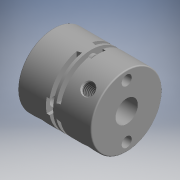
# Autodesk Inventor part: MCGS16-5-8_b
Saved by Autodesk Inventor 2017.3 (Build 213256000, 256)
## iProperties
Part Number: MCGS16-5-8_b
Material: Generic
Catalog Web Link: www.cadenas.de
Description: MCGS, MCGSLK, MCGSRK, MCGSWK_BODY-Couplings - Standard Torque, Set Screw Type - Single Disk Type
Vendor: MISUMI
Document SubType Name: Modeling
Designer: partserver
Manufacturer: MISUMI
Mass: 2.26083 g
Surface Area: 22.403 cm^2
Volume: 2.26083 cm^3
Density: 1 g/cm^3
Appearance: PSOLRGB-192-192-192
Category: PARTsolutions
Company: MISUMI
Title: MCGS16-5-8
Author: Cadenas PARTsolutions
Comments: Couplings - Standard Torque, Set Screw Type - Single Disk Type
PSOL_IDENT_0: {$CADENAS_DATA\23d-libs\misumi\metric\50_couplings\mcgs.prj},241 {VTYP=3D},{NB=MCGS16-5-8_b},{LINA=M
PSOL_IDENT_1: CGS16-5-8},{NN=MCGS, MCGSLK, MCGSRK, MCGSWK_BODY},{DATE=08.06.2021 06:32:33},{GEOMDATE=28.08.2013 00
PSOL_IDENT_2: :00:00},{VERSION=},{LINEID=1040},{WBVAR=HS,KGHS,DD1,ALT1,LDC,DD2,ALT2,RDC,ALT3,ALT4},{WBNUMERIC=LDC,
PSOL_IDENT_3: RDC}  {NB=MCGS16-5-8_b},{LINA=MCGS16-5-8},{KT=DUMMY},{PN=MCGS16-5-8},{HS=MCGS},{HSALG='MCGS','Standa
PSOL_IDENT_4: rd Hole','','Key Groove Hole'},{KGHS=},{KGHSALG='','N/A'},{MATB=Aluminum Die Casting},{MATD=Polyimid
PSOL_IDENT_5: },{STB=Electroless Nickel Plating},{AC=Set Screw},{D=16},{DDIA=16.000},{D1='4','4','5','5','6','6','
PSOL_IDENT_6: 6.35','6.35','7','7','8','8'},{DD1=5},{DD1ALG1='4','4','5','5','6','6','6.35','6.35','7','7','8','8'
PSOL_IDENT_7: },{DD1ALG2=5},{ALT1=},{ALT1ALG=},{LDC=0.0},{LDCALG=0},{LDCALG1=},{LK=0},{D2='5','5','6','6','6.35','
PSOL_IDENT_8: 6.35','7','7','8','8'},{DD2=8},{DDD1=0},{DD2ALG1='5','5','6','6','6.35','6.35','7','7','8','8'},{DD2
PSOL_IDENT_9: ALG11='4','4','5','5','6','6','6.35','6.35','7','7','8','8'},{DD2ALG2=8},{ALT2=},{ALT2ALG=},{RDC=0.0
PSOL_IDENT_10: },{RDCALG=0},{RDCALG1=},{RK=0},{DD3=6.8},{L=16.5},{L1=16.500},{LL=7},{LL1=7.000},{F=3},{F1=3.000},{M=
PSOL_IDENT_11: M3},{T=0.7},{NO=3},{DDIA2=11.2014},{SC1=1.7500},{SC2=6.0000},{DL=5},{TSIMD=3.000},{DR=8},{TSIMIN=2.4
PSOL_IDENT_12: 59},{ALTALG2='','Select RDC'},{TSI=M3},{R1=2.250},{DDIA3=12.000},{LL2=0.950},{C=3.000},{B=3.500},{E=
PSOL_IDENT_13: 3.200},{F2=0.650},{LL3=4.400},{DDIA4=9.000},{TSIMD1=4.800},{TTL=0.0},{TTR=0.0},{ALT3=},{ALT3ALG= '',
PSOL_IDENT_14: 'N/A'},{ALT3PN=},{ALT4=},{ALT4ALG= '', 'N/A'},{ALT4PN=},{KLH=0},{KRH=2},{TTKLH=0.0},{TTKRH=1.0},{MS
PSOL_IDENT_15: S=3},{LSS=4},{DID=7.6}
NB: MCGS16-5-8_b
NN: MCGS, MCGSLK, MCGSRK, MCGSWK_BODY
NT: Couplings - Standard Torque, Set Screw Type - Single Disk Type
NBSYN: $PN._b
LINA: MCGS16-5-8
CATALOG: Misumi
PN: MCGS16-5-8
HS: Standard Hole
KGHS: N/A
MATB: Aluminum Die Casting
MATD: Polyimid
STB: Electroless Nickel Plating
AC: Set Screw
D: 16
DD1: 5
ALT1: w/o LDC (Shaft Hole Diameter Left Shaft)
LDC: 0
DD2: 8
ALT2: w/o RDC (Shaft Hole Diameter Right Shaft)
RDC: 0
L: 16.5
LL: 7
F: 3
M: M3
T: 0.7
ALT3: N/A
ALT4: N/A
SUPPLIER: MISUMI
ARTICLENO: MCGS16-5-8_b
BOMINFO: MCGS16-5-8
CREATOR: CADENAS GmbH
Autodesk Inventor part; units mm, degrees
sketch "Sketch_1" plane through (0, 0, 0) normal (0, 0, 1) x (1, 0, 0)
  line L0 (16.5, 0) -> (0, 0)
  line L1 (0, 7.75) -> (0, 2.5)
  line L2 (0, 2.5) -> (7, 2.5)
  line L3 (7, 2.5) -> (7, 4)
  line L4 (7, 4) -> (7.95, 4)
  line L5 (7.95, 4) -> (7.95, 3.8)
  line L6 (7.95, 3.8) -> (8.55, 3.8)
  line L7 (8.55, 3.8) -> (8.55, 4)
  line L8 (8.55, 4) -> (16.5, 4)
  line L9 (16.5, 4) -> (16.5, 7.75)
  arc A0 (16.5, 7.75) -> (16.25, 8) centre (16.25, 7.75) ccw
  line L10 (16.25, 8) -> (0.25, 8)
  arc A1 (0.25, 8) -> (0, 7.75) centre (0.25, 7.75) ccw
  constraints: 22 end point, 4 point on circle, 2 centre point
revolve "Revolution1" add sketch "Sketch_1" angle 360 about axis through (16.5, 0, 0) along (1, 0, 0)
sketch "Sketch_6" plane through (3, 0, 0) normal (1, 0, 0) x (0, 0, -1)
  line L0 (-1.4142, -1.4142) -> (-5.6569, -5.6569)
  line L1 (-5.6569, -5.6569) -> (-6.7175, -4.5962)
  line L2 (-6.7175, -4.5962) -> (-6.335, -4.5962)
  line L3 (-6.335, -4.5962) -> (-2.2836, -0.5448)
  line L4 (-2.2836, -0.5448) -> (-1.4142, -1.4142)
  line L5 (-1.4142, -1.4142) -> (-5.6569, -5.6569)
  constraints: 12 end point
revolve "Revolution2" cut sketch "Sketch_6" angle 360 about axis through (3, -1.4142, 1.4142) along (0, 0.7071, -0.7071)
thread "Thread1" size "M3x0.5" class "6H" standard "ISO Metric profile" length 5.2295
sketch "Sketch_4" plane through (3, 0, 0) normal (1, 0, 0) x (0, 0, -1)
  line L0 (1.4142, -1.4142) -> (5.6569, -5.6569)
  line L1 (5.6569, -5.6569) -> (4.5962, -6.7175)
  line L2 (4.5962, -6.7175) -> (4.5962, -6.335)
  line L3 (4.5962, -6.335) -> (0.5448, -2.2836)
  line L4 (0.5448, -2.2836) -> (1.4142, -1.4142)
  line L5 (1.4142, -1.4142) -> (5.6569, -5.6569)
  constraints: 12 end point
revolve "Revolution3" cut sketch "Sketch_4" angle 360 about axis through (3, -1.4142, -1.4142) along (0, 0.7071, 0.7071)
thread "Thread2" size "M3x0.5" class "6H" standard "ISO Metric profile" length 5.2295
sketch "Sketch_7" plane through (13.5, 0, 0) normal (1, 0, 0) x (0, 0, -1)
  line L0 (0, 0) -> (-5.6569, -5.6569)
  line L1 (-5.6569, -5.6569) -> (-6.7175, -4.5962)
  line L2 (-6.7175, -4.5962) -> (-6.335, -4.5962)
  line L3 (-6.335, -4.5962) -> (-0.8694, 0.8694)
  line L4 (-0.8694, 0.8694) -> (0, 0)
  line L5 (0, 0) -> (-5.6569, -5.6569)
  constraints: 12 end point
revolve "Revolution4" cut sketch "Sketch_7" angle 360 about axis through (13.5, 0, 0) along (0, 0.7071, -0.7071)
thread "Thread3" size "M3x0.5" class "6H" standard "ISO Metric profile" length 3.7295
sketch "Sketch_5" plane through (13.5, 0, 0) normal (1, 0, 0) x (0, 0, -1)
  line L0 (0, 0) -> (-5.6569, 5.6569)
  line L1 (-5.6569, 5.6569) -> (-4.5962, 6.7175)
  line L2 (-4.5962, 6.7175) -> (-4.5962, 6.335)
  line L3 (-4.5962, 6.335) -> (0.8694, 0.8694)
  line L4 (0.8694, 0.8694) -> (0, 0)
  line L5 (0, 0) -> (-5.6569, 5.6569)
  constraints: 12 end point
revolve "Revolution5" cut sketch "Sketch_5" angle 360 about axis through (13.5, 0, 0) along (0, -0.7071, -0.7071)
thread "Thread4" size "M3x0.5" class "6H" standard "ISO Metric profile" length 3.7295
sketch "Sketch_2" plane through (0, 0, 0) normal (0, 0, 1) x (1, 0, 0)
  line L0 (8.55, 1.5) -> (9.5, 1.75)
  line L1 (9.5, 1.75) -> (9.5, 8)
  line L2 (9.5, 8) -> (8.55, 8)
  line L3 (8.55, 8) -> (8.55, 1.5)
  constraints: 8 end point
extrude "Extrusion1" cut sketch "Sketch_2" along normal mid plane 16
sketch "Sketch_3" plane through (0, 0, 0) normal (0, 0, 1) x (1, 0, 0)
  line L0 (8.55, -1.5) -> (8.55, -8)
  line L1 (8.55, -8) -> (9.5, -8)
  line L2 (9.5, -8) -> (9.5, -1.75)
  line L3 (9.5, -1.75) -> (8.55, -1.5)
  constraints: 8 end point
extrude "Extrusion2" cut sketch "Sketch_3" along normal mid plane 16
sketch "Sketch_16" plane through (0, 0, 0) normal (0, 1, 0) x (-1, 0, 0)
  line L0 (-7, -1.75) -> (-7.95, -1.5)
  line L1 (-7.95, -1.5) -> (-7.95, -8)
  line L2 (-7.95, -8) -> (-7, -8)
  line L3 (-7, -8) -> (-7, -1.75)
  constraints: 8 end point
extrude "Extrusion3" cut sketch "Sketch_16" along normal mid plane 16
sketch "Sketch_17" plane through (0, 0, 0) normal (0, 1, 0) x (-1, 0, 0)
  line L0 (-7, 1.75) -> (-7, 8)
  line L1 (-7, 8) -> (-7.95, 8)
  line L2 (-7.95, 8) -> (-7.95, 1.5)
  line L3 (-7.95, 1.5) -> (-7, 1.75)
  constraints: 8 end point
extrude "Extrusion4" cut sketch "Sketch_17" along normal mid plane 16
sketch "Sketch_18" plane through (7, 0, 0) normal (1, 0, 0) x (0, 0, -1)
  line L0 (-8, 1.6) -> (-8, -1.6)
  line L1 (-8, -1.6) -> (-6, -1.6)
  arc A0 (-6, -1.6) -> (-6, 1.6) centre (-6, 0) ccw
  line L2 (-6, 1.6) -> (-8, 1.6)
  constraints: 6 end point, 2 point on circle, 1 centre point
extrude "Extrusion5" cut sketch "Sketch_18" against normal blind 0.65
sketch "Sketch_19" plane through (7, 0, 0) normal (1, 0, 0) x (0, 0, -1)
  arc A0 (6, 1.6) -> (6, -1.6) centre (6, 0) ccw
  line L0 (6, -1.6) -> (8, -1.6)
  line L1 (8, -1.6) -> (8, 1.6)
  line L2 (8, 1.6) -> (6, 1.6)
  constraints: 6 end point, 2 point on circle, 1 centre point
extrude "Extrusion6" cut sketch "Sketch_19" against normal blind 0.65
sketch "Sketch_20" plane through (9.5, 0, 0) normal (1, 0, 0) x (0, 0, -1)
  arc A0 (-1.6, 6) -> (1.6, 6) centre (0, 6) ccw
  line L0 (1.6, 6) -> (1.6, 8)
  line L1 (1.6, 8) -> (-1.6, 8)
  line L2 (-1.6, 8) -> (-1.6, 6)
  constraints: 6 end point, 2 point on circle, 1 centre point
extrude "Extrusion7" cut sketch "Sketch_20" along normal blind 0.65
sketch "Sketch_21" plane through (9.5, 0, 0) normal (1, 0, 0) x (0, 0, -1)
  line L0 (-1.6, -6) -> (-1.6, -8)
  line L1 (-1.6, -8) -> (1.6, -8)
  line L2 (1.6, -8) -> (1.6, -6)
  arc A0 (1.6, -6) -> (-1.6, -6) centre (0, -6) ccw
  constraints: 6 end point, 2 point on circle, 1 centre point
extrude "Extrusion8" cut sketch "Sketch_21" along normal blind 0.65
sketch "Sketch_22" plane through (7.95, 0, 0) normal (1, 0, 0) x (0, 0, -1)
  circle A0 centre (-6, 0) radius 1.2375
  constraints: 1 centre point
extrude "Extrusion9" add sketch "Sketch_22" against normal blind 0.65
sketch "Sketch_23" plane through (7.95, 0, 0) normal (1, 0, 0) x (0, 0, -1)
  circle A0 centre (6, 0) radius 1.2375
  constraints: 1 centre point
extrude "Extrusion10" add sketch "Sketch_23" against normal blind 0.65
sketch "Sketch_24" plane through (8.55, 0, 0) normal (1, 0, 0) x (0, 0, -1)
  circle A0 centre (0, 6) radius 1.2375
  constraints: 1 centre point
extrude "Extrusion11" add sketch "Sketch_24" along normal blind 0.65
sketch "Sketch_25" plane through (8.55, 0, 0) normal (1, 0, 0) x (0, 0, -1)
  circle A0 centre (0, -6) radius 1.2375
  constraints: 1 centre point
extrude "Extrusion12" add sketch "Sketch_25" along normal blind 0.65
sketch "Sketch18" plane through (0, 0, 0) normal (-1, 0, 0) x (0, 0, 1)
  point P0 (-6, 0)
hole "Hole1" at (0, 0, -6) direction (1, 0, 0) diameter 2.25 depth 7
sketch "Sketch19" plane through (0, 0, 0) normal (-1, 0, 0) x (0, 0, 1)
  point P0 (6, 0)
hole "Hole2" at (0, 0, 6) direction (1, 0, 0) diameter 2.25 depth 7
sketch "Sketch20" plane through (16.5, 0, 0) normal (1, 0, 0) x (0, 0, -1)
  point P0 (0, 6)
hole "Hole3" at (16.5, 6, 0) direction (-1, 0, 0) diameter 2.25 depth 7
sketch "Sketch21" plane through (16.5, 0, 0) normal (1, 0, 0) x (0, 0, -1)
  point P0 (0, -6)
hole "Hole4" at (16.5, -6, 0) direction (-1, 0, 0) diameter 2.25 depth 7
ref_plane "to_screw1_XY" through (3, -5.6569, 5.6569) normal (0, -0.7071, 0.7071) x (1, 0, 0)
ref_plane "to_screw1_YZ" through (3, -5.6569, 5.6569) normal (1, 0, 0) x (0, 0.7071, 0.7071)
ref_plane "to_screw1_ZX" through (3, -5.6569, 5.6569) normal (0, 0.7071, 0.7071) x (0, -0.7071, 0.7071)
ref_plane "to_screw2_XY" through (13.5, -5.6569, 5.6569) normal (0, -0.7071, 0.7071) x (1, 0, 0)
ref_plane "to_screw2_YZ" through (13.5, -5.6569, 5.6569) normal (1, 0, 0) x (0, 0.7071, 0.7071)
ref_plane "to_screw2_ZX" through (13.5, -5.6569, 5.6569) normal (0, 0.7071, 0.7071) x (0, -0.7071, 0.7071)
ref_plane "to_screw3_XY" through (13.5, 5.6569, 5.6569) normal (0, 0.7071, 0.7071) x (1, 0, 0)
ref_plane "to_screw3_YZ" through (13.5, 5.6569, 5.6569) normal (1, 0, 0) x (0, 0.7071, -0.7071)
ref_plane "to_screw3_ZX" through (13.5, 5.6569, 5.6569) normal (0, 0.7071, -0.7071) x (0, 0.7071, 0.7071)
ref_plane "to_screw4_XY" through (3, -5.6569, -5.6569) normal (0, 0.7071, 0.7071) x (1, 0, 0)
ref_plane "to_screw4_YZ" through (3, -5.6569, -5.6569) normal (1, 0, 0) x (0, 0.7071, -0.7071)
ref_plane "to_screw4_ZX" through (3, -5.6569, -5.6569) normal (0, 0.7071, -0.7071) x (0, 0.7071, 0.7071)
body "Solid1"
